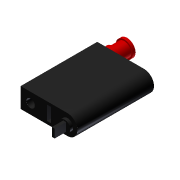
# Autodesk Inventor part: Vacuum Valve 1764
Saved by Autodesk Inventor 2011 (Build 150239000, 239)
## iProperties
Created: 2010-02-15
Part Number: Vacuum Valve 1764
Document SubType Name: Modeling
Designer: jgehrig
Density: 1 g/cm^3
Author: jgehrig
Autodesk Inventor part; units mm, degrees
ref_plane "YZ Plane" through (0, 0, 0) normal (1, 0, 0) x (0, 1, 0)
ref_plane "XZ Plane" through (0, 0, 0) normal (0, 1, 0) x (-1, 0, 0)
ref_plane "XY Plane" through (0, 0, 0) normal (0, 0, 1) x (1, 0, 0)
sketch "Sketch1" plane through (0, 0, 0) normal (0, 0, 1) x (1, 0, 0)
  line L0 (-20.4019, 15.1575) -> (4.9981, 15.1575)
  line L1 (4.9981, 15.1575) -> (4.9981, 6.2675)
  line L2 (4.9981, 6.2675) -> (-20.4019, 6.2675)
  line L3 (-20.4019, 6.2675) -> (-20.4019, 15.1575)
  arc A0 (0.5531, 6.2675) -> (0.5531, 15.1575) centre (0.5531, 10.7125) ccw
  circle A1 centre (-15.9569, 10.7125) radius 1.905
  circle A2 centre (0.5531, 10.7125) radius 1.905
  line L4 (-8.6544, 13.8875) -> (-6.7494, 13.8875)
  line L5 (-6.7494, 13.8875) -> (-6.7494, 7.5375)
  line L6 (-6.7494, 7.5375) -> (-8.6544, 7.5375)
  line L7 (-8.6544, 7.5375) -> (-8.6544, 13.8875)
  point P0 (0, 0)
  dimension "d0" = 25.4
  dimension "d1" = 8.89
  dimension "d2" = 0
  dimension "d3" = 0
  dimension "d4" = 3.81
  dimension "d5" = 3.81
  dimension "d6" = 0
  dimension "d7" = 4.445
  dimension "d8" = 4.445
  dimension "d9" = 7.3025
  dimension "d12" = 1.905
  dimension "d13" = 6.35
  constraints: 16 end point, 4 parallel, 3 centre point, 2 horizontal, 2 perpendicular, 2 point on circle, 2 point on line, 1 tangent
  measures "d0" distance of L0.start L0.end
  measures "d1" distance of L2.end L0.start
  measures "d2" horizontal distance of A0.end A0.centre
  measures "d3" horizontal distance of A0.centre A0.start
  measures "d4" diameter of A1
  measures "d5" diameter of A2
  measures "d6" distance of A0.centre A2.centre
  measures "d7" distance from line of L3 A1.centre
  measures "d8" distance from line of L1 A0.centre
  measures "d9" distance from line of A1.centre L7
  measures "d12" distance of L5.end L6.end
  measures "d13" distance of L6.end L4.start
extrude "Extrusion1" add sketch "Sketch1" along normal blind 34.29 contours L0 A0 L2 L3
sketch "Sketch2" plane through (0, 0, 0) normal (0, 0, -1) x (-1, 0, 0)
  circle A0 centre (15.9569, 10.7125) radius 1.905 projected
  circle A1 centre (15.9569, 10.7125) radius 1.905
  circle A2 centre (15.9569, 10.7125) radius 3.81
  point P0 (0, 0)
  dimension "d19" = 7.62
  constraints: 2 centre point, 2 coincident, 1 concentric
  measures "d19" diameter of A2
extrude "Extrusion2" add sketch "Sketch2" along normal blind 2.54 contours A0 | A2
sketch "Sketch3" plane through (-15.9569, 10.7125, -2.54) normal (0, 0, -1) x (-1, 0, 0)
  circle A0 centre (0, 0) radius 3.81 projected
  circle A1 centre (0, 0) radius 3.175
  point P0 (-15.9569, -10.7125)
  dimension "d22" = 6.35
  constraints: 1 centre point, 1 coincident
  measures "d22" diameter of A1
extrude "Extrusion3" add sketch "Sketch3" along normal blind 5.08 contours A1
sketch "Sketch4" plane through (-15.9569, 10.7125, -7.62) normal (0, 0, -1) x (-1, 0, 0)
  circle A0 centre (0, 0) radius 3.81 projected
  circle A1 centre (0, 0) radius 3.81
  point P0 (-15.9569, -10.7125)
  constraints: 1 centre point, 1 coincident, 1 concentric
extrude "Extrusion4" add sketch "Sketch4" along normal blind 1.27
sketch "Sketch5" plane through (0, 0, 34.29) normal (0, 0, 1) x (1, 0, 0)
  arc A0 (0.5531, 6.2675) -> (0.5531, 15.1575) centre (0.5531, 10.7125) ccw projected
  circle A1 centre (0.5531, 10.7125) radius 2.54
  point P0 (0, 0)
  dimension "d27" = 5.08
  constraints: 1 centre point, 1 coincident
  measures "d27" diameter of A1
extrude "Extrusion5" add sketch "Sketch5" along normal blind 1.27
sketch "Sketch6" plane through (0.5531, 10.7125, 35.56) normal (0, 0, 1) x (1, 0, 0)
  circle A0 centre (0, 0) radius 2.54 projected
  line L0 (-0.635, 1.905) -> (0.635, 1.905)
  line L1 (0.635, 1.905) -> (0.635, -1.905)
  line L2 (0.635, -1.905) -> (-0.635, -1.905)
  line L3 (-0.635, -1.905) -> (-0.635, 1.905)
  point P0 (-0.5531, -10.7125)
  dimension "d30" = 3.81
  dimension "d31" = 1.27
  dimension "d32" = 0.635
  dimension "d33" = 1.905
  constraints: 8 end point, 2 parallel, 1 horizontal, 1 perpendicular
  measures "d30" distance of L0.end L1.end
  measures "d31" distance of L1.end L2.end
  measures "d32" distance from line of L3 A0.centre
  measures "d33" distance from line of A0.centre L0
extrude "Extrusion6" add sketch "Sketch6" along normal blind 5.08 contours L0 L1 L2 L3
body "Solid1"
